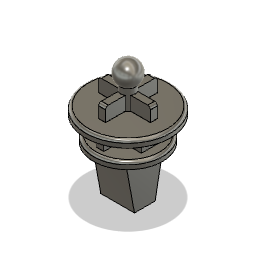
ford-focus-mk1-hatchback-parcel-shelf-hanger-clip-v1 (Autodesk Fusion 360 design; units mm, degrees)
Autodesk Fusion 360 part; units mm, degrees
sketch "Sketch1" plane through (0, 0, 0) normal (0, 1, 0) x (1, 0, 0)
  line L0 (4.875, 3) -> (-4.875, 3)
  line L1 (-4.875, 3) -> (-4.875, -3)
  line L2 (-4.875, -3) -> (4.875, -3)
  line L3 (4.875, -3) -> (4.875, 3)
  line L4 (4.875, 3) -> (-4.875, -3) construction
  line L5 (-4.875, 3) -> (4.875, -3) construction
  dimension "d1" = 9.75
  dimension "d2" = 6
  constraint horizontal L0
  constraint perpendicular L0 L1
  constraint parallel L0 L2
  constraint parallel L1 L3
  constraint coincident L4 origin
  constraint coincident L5 origin
  measures "d1" distance of L1.end L2.end
  measures "d2" distance of L0.start L2.end
extrude "Extrude1" add sketch "Sketch1" along normal blind 12 makes body 1
draft "Draft1" angle 10.5 neutral plane through (0, 0, 0) pull (0, -1, 0) 1 faces at (-1.625, 4, 3) on bodies 1
draft "Draft2" angle 10.5 neutral plane through (0, 0, 0) pull (0, -1, 0) 1 faces at (1.625, 4, -3) on bodies 1
sketch "Sketch2" plane through (0, 12, 0) normal (0, 1, 0) x (-1, 0, 0)
  line L0 (-4.875, 5.2241) -> (-4.875, -5.2241)
  line L1 (4.875, -5.2241) -> (4.875, 5.2241)
  line L2 (-4.875, -5.2241) -> (4.875, -5.2241)
  line L3 (4.875, 5.2241) -> (-4.875, 5.2241)
  line L4 (4.875, 3) -> (-4.875, 3)
  line L5 (-4.875, 3) -> (-4.875, -3)
  line L6 (-4.875, -3) -> (4.875, -3)
  line L7 (4.875, -3) -> (4.875, 3)
  line L8 (4.875, 3) -> (-4.875, -3) construction
  line L9 (-4.875, 3) -> (4.875, -3) construction
  dimension "d11" = 6
  dimension "d12" = 9.75
  constraint horizontal L4
  constraint perpendicular L4 L5
  constraint parallel L4 L6
  constraint parallel L5 L7
  constraint coincident L8 origin
  constraint coincident L9 origin
  measures "d11" distance of L4.end L5.end
  measures "d12" distance of L4.start L4.end
extrude "Extrude2" add sketch "Sketch2" along normal blind 2 contours L0 L1 L4 L5 L6 L7 bodies 1
sketch "Sketch3" plane through (0, 14, 0) normal (0, 1, 0) x (-1, 0, 0)
  line L0 (4.875, -3) -> (4.875, 3)
  line L1 (4.875, 3) -> (-4.875, 3)
  line L2 (-4.875, 3) -> (-4.875, -3)
  line L3 (-4.875, -3) -> (4.875, -3)
  circle A0 centre (0, 0) radius 10
  dimension "d15" = 20
  constraint coincident A0.centre origin
  measures "d15" diameter of A0
extrude "Extrude3" add sketch "Sketch3" along normal blind 2 separate body makes body 2
extrude "Extrude4" add 1 faces at (1.625, 14, 1) along direction (0, 1, 0) blind 7 on bodies 1 bodies 1 2
sketch "Sketch4" plane through (0, 21, 0) normal (0, 1, 0) x (-1, 0, 0)
  line L0 (4.875, -3) -> (4.875, 3)
  line L1 (4.875, 3) -> (-4.875, 3)
  line L2 (-4.875, 3) -> (-4.875, -3)
  line L3 (-4.875, -3) -> (4.875, -3)
  circle A0 centre (0, 0) radius 12.25
  dimension "d20" = 24.5
  constraint coincident A0.centre origin
  measures "d20" diameter of A0
extrude "Extrude5" add sketch "Sketch4" along normal blind 2 contours L0 L1 L2 L3 | A0 bodies 1
sketch "Sketch5" plane through (0, 0, 3) normal (0, 0, 1) x (1, 0, 0)
  line L0 (-4.875, 16) -> (4.875, 16)
  line L1 (4.875, 16) -> (4.875, 21)
  line L2 (4.875, 21) -> (-4.875, 21)
  line L3 (-4.875, 21) -> (-4.875, 16)
  line L4 (0.9958, 22) -> (-1.0042, 22)
  line L5 (-1.0042, 22) -> (-1.0042, 15)
  line L6 (-1.0042, 15) -> (0.9958, 15)
  line L7 (0.9958, 15) -> (0.9958, 22)
  line L8 (0.9958, 22) -> (-1.0042, 15) construction
  line L9 (-1.0042, 22) -> (0.9958, 15) construction
  point P0 (-0.0042, 18.5)
  dimension "d23" = 2
  dimension "d42" = 7
  constraint horizontal L4
  constraint perpendicular L4 L5
  constraint parallel L4 L6
  constraint parallel L5 L7
  constraint coincident L8 P0
  constraint coincident L9 P0
  measures "d23" distance of L5.end L6.end
  measures "d42" distance of L4.end L5.end
extrude "Extrude6" add sketch "Sketch5" along normal blind 5 and the other way blind 11 contours L0 L2 L5 L7 bodies 1
sketch "Sketch7" plane through (0, 23, 0) normal (0, 1, 0) x (-1, 0, 0)
  circle A0 centre (0, 0) radius 12.25
  line L0 (-7.5, 1) -> (-7.5, -1)
  line L1 (7.5, -1) -> (7.5, 1)
  line L2 (7.5, 1) -> (-7.5, -1) construction
  line L3 (-7.5, 1) -> (7.5, -1) construction
  line L4 (1, 7.5) -> (-1, 7.5)
  line L5 (-1, -7.5) -> (1, -7.5)
  line L6 (1, 7.5) -> (-1, -7.5) construction
  line L7 (-1, 7.5) -> (1, -7.5) construction
  line L8 (1, -1) -> (7.5, -1)
  line L9 (-7.5, -1) -> (-1, -1)
  line L10 (-1, 1) -> (-7.5, 1)
  line L11 (7.5, 1) -> (1, 1)
  line L12 (1, -7.5) -> (1, -1)
  line L13 (1, 1) -> (1, 7.5)
  line L14 (-1, -1) -> (-1, -7.5)
  line L15 (-1, 7.5) -> (-1, 1)
  dimension "d28" = 2
  dimension "d29" = 15
  dimension "d30" = 15
  dimension "d31" = 2
  constraint horizontal L11
  constraint perpendicular L0 L11
  constraint parallel L9 L11
  constraint parallel L0 L1
  constraint coincident L2 A0.centre
  constraint coincident L3 A0.centre
  constraint coincident A0.centre origin
  constraint horizontal L4
  constraint perpendicular L4 L15
  constraint parallel L4 L5
  constraint parallel L12 L15
  constraint coincident L6 A0.centre
  constraint coincident L7 A0.centre
  constraint collinear L8 L9
  constraint coincident L9.end L15
  constraint collinear L10 L11
  constraint coincident L11.end L12
  constraint collinear L12 L13
  constraint collinear L14 L15
  measures "d28" distance of L0.start L0.end
  measures "d29" distance of L0.end L1.start
  measures "d30" distance of L4.end L5.start
  measures "d31" distance of L5.start L5.end
extrude "Extrude7" add sketch "Sketch7" along normal blind 4 contours L0 L1 L4 L5 L8 L9 L10 L11 L12 L13 L14 L15 bodies 1
sketch "Sketch8" plane through (0, 27, 0) normal (0, 1, 0) x (-1, 0, 0)
  line L0 (-1, 7.5) -> (-1, 1)
  line L1 (-1, 1) -> (-7.5, 1)
  line L2 (-7.5, 1) -> (-7.5, -1)
  line L3 (-7.5, -1) -> (-1, -1)
  line L4 (-1, -1) -> (-1, -7.5)
  line L5 (-1, -7.5) -> (1, -7.5)
  line L6 (1, -7.5) -> (1, -1)
  line L7 (1, -1) -> (7.5, -1)
  line L8 (7.5, -1) -> (7.5, 1)
  line L9 (7.5, 1) -> (1, 1)
  line L10 (1, 1) -> (1, 7.5)
  line L11 (1, 7.5) -> (-1, 7.5)
  circle A0 centre (0, 0) radius 2.1
  dimension "d34" = 4.2
  constraint coincident A0.centre origin
  measures "d34" diameter of A0
extrude "Extrude8" add sketch "Sketch8" along normal blind 4.4 and the other way blind 5 contours L0 L1 L3 L4 L6 L7 L9 L10 A0 | L0 L1 A0 | L9 L10 A0 | L3 L4 A0 | L6 L7 A0 bodies 1
sphere "SpherePrimitive1" add diameter 6.8 placed x (-1, 0, 0) y (0, 0, 1) z (0, 1, 0) at (0, 31.4, 0) bodies 1
fillet "Fillet2" radius 0.8 6 edges at (7.5, 27, 0) (0, 27, 7.5) (0, 27, -7.5) (-7.5, 27, 0) (11.421, 23, -4.4298) (9.3233, 16, -3.6162) on bodies 1
extrude "Extrude9" add 1 faces at (4.875, 17.6667, 1) along direction (1, 0, 0) blind -12 and the other way blind -2 on bodies 1 bodies 1
